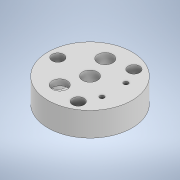
# Autodesk Inventor part: water
Saved by Autodesk Inventor 2020 (Build 240168000, 168)
## iProperties
Created: 2019-06-21
Part Number: water
Material: Generic
Document SubType Name: Modeling
Designer: ColinP
Density: 1 g/cm^3
Appearance: Default
Mass: 2.35354 g
Surface Area: 74.254 cm^2
Volume: 2.35354 cm^3
Author: ColinP
Autodesk Inventor part; units mm, degrees
ref_plane "YZ Plane" through (0, 0, 0) normal (1, 0, 0) x (0, 1, 0)
ref_plane "XZ Plane" through (0, 0, 0) normal (0, 1, 0) x (-1, 0, 0)
ref_plane "XY Plane" through (0, 0, 0) normal (0, 0, 1) x (1, 0, 0)
sketch "Sketch1" plane through (0, 0, 0) normal (0, 1, 0) x (-1, 0, 0)
  circle A0 centre (0, 0) radius 17.78
  dimension "d0" = 35.56
  constraints: 1 centre point, 1 coincident
  measures "d0" diameter of A0
extrude "Extrusion1" add sketch "Sketch1" along normal blind 10.16
sketch "Sketch2" plane through (0, 10.16, 0) normal (0, 1, 0) x (1, 0, 0)
  circle A0 centre (0, 0) radius 17.78 projected
  constraints: 1 coincident
hole "Hole1" at (0, 10.16, 0) direction (0, -1, 0) diameter 6.35 end through all
sketch "Sketch3" plane through (0, 10.16, 0) normal (0, 1, 0) x (1, 0, 0)
  line L0 (0, 0) -> (-13.6144, 0)
  dimension "d10" = 13.6144
  constraints: 2 end point, 1 horizontal
  measures "d10" distance of L0.start L0.end
hole "Hole2" at (-13.6144, 10.16, 0) direction (0, -1, 0) diameter 4.9022 end through all
pattern_circular "Circular Pattern1" count 3 over 360 about axis through (0, -41.1455, 0) along (0, 1, 0) of "Hole2"
sketch "Sketch23" plane through (0, 10.16, 0) normal (0, 1, 0) x (1, 0, 0)
  line L0 (0, 0) -> (10.16, 0)
  line L1 (10.16, 0) -> (10.16, 5.08)
  line L2 (10.16, 5.08) -> (10.16, -5.08)
  dimension "d122" = 10.16
  dimension "d123" = 5.08
  dimension "d124" = 10.16
  constraints: 6 end point, 1 horizontal, 1 perpendicular, 1 point on line
  measures "d122" distance of L0.start L0.end
  measures "d123" distance of L0.end L1.end
  measures "d124" distance of L1.end L2.end
hole "Hole10" at (10.16, 10.16, -5.08) at (10.16, 10.16, 5.08) direction (0, -1, 0) diameter 1.905 end through all
shell "Shell4" thickness 0.635 removed faces 0
sketch "Sketch26" plane through (0, 10.16, 0) normal (0, 1, 0) x (1, 0, 0)
  line L0 (0, 0) -> (-3.175, 9.6512)
  line L1 (-3.175, 9.6512) -> (0, 0)
  line L2 (0, 0) -> (-3.175, -9.6512)
  dimension "d148" = 10.16
  dimension "d149" = 10.16
  constraints: 6 end point, 1 collinear
  measures "d148" distance of L0.start L0.end
  measures "d149" distance of L0.start L2.end
hole "Hole12" at (-3.175, 10.16, -9.6512) at (-3.175, 10.16, 9.6512) direction (0, -1, 0) diameter 6.35 depth 2.54
sketch "Sketch27" plane through (0, 10.16, 0) normal (0, 1, 0) x (1, 0, 0)
  circle A0 centre (-3.175, 9.6512) radius 3.175 projected
  circle A1 centre (-3.175, 9.6512) radius 3.81
  circle A2 centre (-3.175, -9.6512) radius 3.175 projected
  circle A3 centre (-3.175, -9.6512) radius 3.81
  point P0 (0, 0)
  dimension "d157" = 7.62
  dimension "d158" = 7.62
  constraints: 2 centre point, 2 coincident
  measures "d157" diameter of A1
  measures "d158" diameter of A3
extrude "Extrusion15" add sketch "Sketch27" against normal blind 5.08 contours A1
extrude "Extrusion16" add sketch "Sketch27" against normal blind 2.54 contours A3
body "Solid1"
